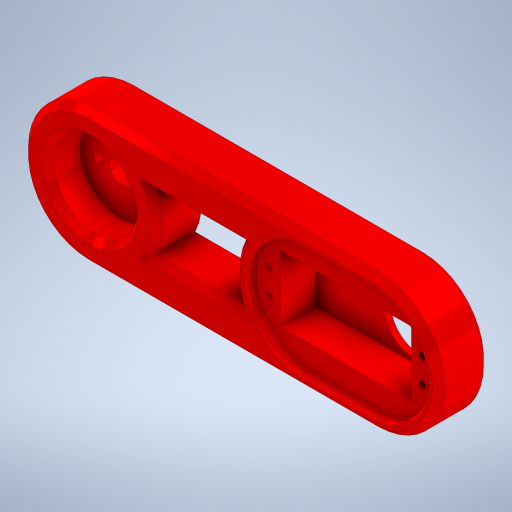
# Autodesk Inventor part: arm_part2
Saved by Autodesk Inventor 2023 (Build 270158000, 158)
## iProperties
Created: 2023-01-15
Part Number: arm_part2
Material: PLA plastic
Document SubType Name: Modeling
Designer: denyh
Density: 1.25 g/cm^3
Appearance: Generic
Author: denyh
Autodesk Inventor part; units mm, degrees
ref_plane "YZ Plane" through (0, 0, 0) normal (1, 0, 0) x (0, 1, 0)
ref_plane "XZ Plane" through (0, 0, 0) normal (0, 1, 0) x (-1, 0, 0)
ref_plane "XY Plane" through (0, 0, 0) normal (0, 0, 1) x (1, 0, 0)
sketch "Sketch2" plane through (0, 0, 0) normal (0, 0, 1) x (1, 0, 0)
  circle A0 centre (0, 0) radius 21
  line L0 (0, 0) -> (88, 0)
  circle A1 centre (88, 0) radius 21
  line L1 (0, 21) -> (88, 21)
  line L2 (0, -21) -> (88, -21)
  line L3 (0, 0) -> (24, 0)
  line L4 (88, 0) -> (64, 0)
  point P0 (67, 9)
  point P1 (67, -9)
  dimension "d1" = 42
  dimension "d2" = 88
  dimension "d3" = 42
  dimension "d4" = 24
  dimension "d6" = 24
  constraints: 10 end point, 4 point on circle, 2 centre point, 2 coincident, 2 horizontal, 2 point on line, 2 tangent
  measures "d1" diameter of A0
  measures "d2" distance of L0.start L0.end
  measures "d3" diameter of A1
  measures "d4" distance of L0.start L3.end
  measures "d6" distance of L4.start L4.end
extrude "Extrusion1" add sketch "Sketch2" along normal blind 16
sketch "Sketch3" plane through (0, 0, 16) normal (0, 0, 1) x (1, 0, 0)
  circle A0 centre (0, 0) radius 13
  dimension "d10" = 26
  constraints: 1 centre point, 1 coincident
  measures "d10" diameter of A0
sketch "Sketch4" plane through (0, 0, 16) normal (0, 0, 1) x (1, 0, 0)
  arc A0 (88, -21) -> (88, 21) centre (88, 0) ccw projected
  line L0 (109, 0) -> (107, 0)
  line L1 (104, 0) -> (88, 0)
  line L2 (88, 0) -> (47, 0)
  line L3 (104, 0) -> (96, 0)
  line L4 (107, 0) -> (101, 0)
  line L5 (101, 0) -> (101, 3.9)
  line L6 (101, 3.9) -> (101, -3.9)
  circle A1 centre (101, 3.9) radius 1.1
  circle A2 centre (101, -3.9) radius 1.1
  line L7 (101, 0) -> (97.5, 0)
  line L8 (97.5, 0) -> (97.5, 10.25)
  line L9 (97.5, 10.25) -> (56.5, 10.25)
  line L10 (56.5, 10.25) -> (56.5, -10.25)
  line L11 (56.5, -10.25) -> (97.5, -10.25)
  line L12 (97.5, -10.25) -> (97.5, 0)
  line L13 (56.5, 0) -> (53, 0)
  line L14 (53, 0) -> (53, 3.9)
  circle A3 centre (53, 3.9) radius 1.1
  circle A4 centre (53, -3.9) radius 1.1
  arc A5 (88, -17) -> (88, 17) centre (88, 0) ccw
  line L15 (56.5, 0) -> (66, 0)
  line L16 (66, 17) -> (88, 17)
  line L17 (66, -17) -> (88, -17)
  arc A6 (66, 17) -> (66, -17) centre (66, 0) ccw
  line L18 (97.5, 0) -> (87, 0)
  circle A7 centre (87, 0) radius 9
  point P0 (0, 0)
  dimension "d12" = 2
  dimension "d14" = 41
  dimension "d16" = 6
  dimension "d17" = 3.9
  dimension "d18" = 7.8
  dimension "d19" = 2.2
  dimension "d20" = 2.2
  dimension "d21" = 3.5
  dimension "d22" = 10.25
  dimension "d23" = 41
  dimension "d24" = 20.5
  dimension "d25" = 3.5
  dimension "d26" = 2.2
  dimension "d27" = 34
  dimension "d28" = 9.5
  dimension "d31" = 10.5
  dimension "d32" = 18
  constraints: 38 end point, 8 point on line, 7 centre point, 7 coincident, 7 perpendicular, 5 point on circle, 2 horizontal, 2 midpoint, 1 tangent
  measures "d12" distance of L0.start L0.end
  measures "d14" distance of L1.end L2.end
  measures "d16" distance of L0.end L4.end
  measures "d17" distance of L4.end L5.end
  measures "d18" distance of L5.end L6.end
  measures "d19" diameter of A1
  measures "d20" diameter of A2
  measures "d21" distance of L4.end L7.end
  measures "d22" distance of L7.end L8.end
  measures "d23" distance of L8.end L9.end
  measures "d24" distance of L9.end L10.end
  measures "d25" distance of L13.start L13.end
  measures "d26" diameter of A4
  measures "d27" diameter of A5
  measures "d28" distance of L13.start L15.end
  measures "d31" distance of L7.end L18.end
  measures "d32" diameter of A7
extrude "Extrusion2" cut sketch "Sketch4" against normal blind 3 contours L4 A5 L17 A6 L2 L10 L11 L12 L1 | L1 L8 L9 L10 L2 A6 L16 A5 L4 | L12 L11 L10 L2 A7 L1 | L1 A7 L2 L10 L9 L8 | A7 L2 L1 | L1 L2 A7 | A1 | A2 | A3 | A4
extrude "Extrusion3" cut sketch "Sketch4" against normal blind 14 contours L12 L11 L10 L2 A7 L1 | L1 A7 L2 L10 L9 L8 | A7 L2 L1 | L1 L2 A7
extrude "Extrusion4" cut sketch "Sketch4" against normal blind 20 contours A7 L2 L1 | L1 L2 A7
extrude "Extrusion5" cut sketch "Sketch4" against normal blind 12 contours A1 | A2 | A3 | A4
chamfer "Chamfer1" distance 2 angle 45 4 edges at (44, 21, 16) (-21, 0, 16) (44, -21, 16) (109, 0, 16)
extrude "Extrusion6" cut sketch "Sketch3" against normal blind 10
chamfer "Chamfer2" distance 2 angle 45 1 edges at (-13, 0, 16)
chamfer "Chamfer3" distance 1 angle 45 4 edges at (49, 0, 16) (77, 17, 16) (105, 0, 16) (77, -17, 16)
sketch "Sketch5" plane through (0, 0, 6) normal (0, 0, 1) x (1, 0, 0)
  circle A0 centre (0, 0) radius 3.75
  line L0 (0, 0) -> (7.25, 0)
  circle A1 centre (7.25, 0) radius 1.5
  line L1 (0, 0) -> (-7.25, 0)
  circle A2 centre (-7.25, 0) radius 1.5
  dimension "d52" = 7.5
  dimension "d53" = 7.25
  dimension "d54" = 3
  dimension "d55" = 7.25
  dimension "d56" = 3
  constraints: 4 end point, 3 centre point, 3 coincident, 2 horizontal
  measures "d52" diameter of A0
  measures "d53" distance of L0.start L0.end
  measures "d54" diameter of A1
  measures "d55" distance of L0.start L1.end
  measures "d56" diameter of A2
extrude "Extrusion7" cut sketch "Sketch5" against normal blind 10
chamfer "Chamfer4" distance 2 angle 45 4 edges at (44, -21, 0) (109, 0, 0) (44, 21, 0) (-21, 0, 0)
sketch "Sketch6" plane through (0, 0, 16) normal (0, 0, 1) x (1, 0, 0)
  circle A0 centre (0, 0) radius 21
  arc A1 (66, 17) -> (66, -17) centre (66, 0) ccw projected
  circle A2 centre (66, 0) radius 21
  line L0 (88, 21) -> (0, 21) projected
  line L1 (45, 9) -> (18.9737, 9)
  line L2 (45, 9) -> (47.0263, 9)
  line L3 (18.9737, 9) -> (18.9737, -9)
  line L4 (18.9737, -9) -> (47.0263, -9)
  constraints: 8 end point, 5 point on circle, 2 centre point, 2 coincident, 1 horizontal, 1 perpendicular, 1 vertical
extrude "Extrusion8" cut sketch "Sketch6" against normal blind 105.25 contours A0 L1 L2 A2 L4
chamfer "Chamfer5" distance 2 angle 45 8 edges at (33, 9, 16) (21, 0, 16) (33, -9, 16) (45, 0, 16) (21, 0, 0) (33, -9, 0) (45, 0, 0) (33, 9, 0)
body "Solid1"
